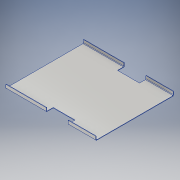
# Autodesk Inventor part: BellyPan
Saved by Autodesk Inventor 2016 (Build 200138000, 138)
## iProperties
Created: 2017-01-21
Part Number: BellyPan
Material: Aluminum 6061
Document SubType Name: Modeling
Designer: hamblettk
Density: 2.7 g/cm^3
Appearance: Aluminum - Flat
Author: hamblettk
Autodesk Inventor part; units mm, degrees
ref_plane "YZ Plane" through (0, 0, 0) normal (1, 0, 0) x (0, 1, 0)
ref_plane "XZ Plane" through (0, 0, 0) normal (0, 1, 0) x (-1, 0, 0)
ref_plane "XY Plane" through (0, 0, 0) normal (0, 0, 1) x (1, 0, 0)
sketch "Sketch2" plane through (0, 0, 0) normal (1, 0, 0) x (0, 1, 0)
  line L0 (0, 0) -> (0, -269.875)
  line L1 (0, 0) -> (0, 269.875)
  line L2 (0, 269.875) -> (25.4, 269.875)
  line L3 (0, -269.875) -> (25.4, -269.875)
  line L4 (25.4, -269.875) -> (25.4, -266.7)
  line L5 (25.4, 269.875) -> (25.4, 266.7)
  line L6 (25.4, 266.7) -> (3.175, 266.7)
  line L7 (25.4, -266.7) -> (3.175, -266.7)
  line L8 (3.175, -266.7) -> (3.175, 266.7)
  dimension "d10" = 269.875
  dimension "d11" = 269.875
  dimension "d12" = 25.4
  dimension "d13" = 25.4
  dimension "d14" = 3.175
  dimension "d15" = 3.175
  dimension "d16" = 22.225
  dimension "d17" = 22.225
  constraints: 18 end point, 4 vertical, 3 horizontal, 1 perpendicular
  measures "d10" distance of L0.start L0.end
  measures "d11" distance of L0.start L1.end
  measures "d12" distance of L1.end L2.end
  measures "d13" distance of L0.end L3.end
  measures "d14" distance of L3.end L4.end
  measures "d15" distance of L2.end L5.end
  measures "d16" distance of L5.end L6.end
  measures "d17" distance of L4.end L7.end
extrude "Extrusion2" add sketch "Sketch2" along normal blind 616.1532
fillet "Fillet1" radius 3.175 4 edges at (308.0766, 0, 269.875) (308.0766, 0, -269.875) (308.0766, 3.175, -266.7) (308.0766, 3.175, 266.7)
sketch "Sketch5" plane through (616.1532, 0, 0) normal (1, 0, 0) x (0, 0, -1)
  arc A0 (-269.875, 3.175) -> (-266.7, 0) centre (-266.7, 3.175) ccw projected
  line L0 (-266.7, 0) -> (-266.7, 3.175)
  line L1 (263.525, 3.175) -> (-263.525, 3.175) projected
  line L2 (-266.7, 3.175) -> (263.525, 3.175)
  line L3 (263.525, 3.175) -> (263.525, 0)
  line L4 (-266.7, 0) -> (266.7, 0) projected
  line L5 (263.525, 0) -> (-266.7, 0)
  point P0 (0, 0)
  constraints: 8 end point, 1 collinear, 1 horizontal, 1 perpendicular, 1 point on line, 1 tangent, 1 vertical
extrude "Extrusion6" add sketch "Sketch5" along normal blind 7.112
sketch "Sketch6" plane through (616.1532, 0, 0) normal (1, 0, 0) x (0, 0, -1)
  line L0 (-266.7, 6.35) -> (-266.7, 25.4) projected
  line L1 (-266.7, 25.4) -> (-269.875, 25.4) projected
  line L2 (-269.875, 25.4) -> (-269.875, 3.175) projected
  line L3 (-266.7, 3.175) -> (-263.525, 3.175) projected
  arc A0 (-266.7, 6.35) -> (-263.525, 3.175) centre (-263.525, 6.35) ccw projected
  line L4 (-266.7, 6.35) -> (-266.7, 25.4) projected
  line L5 (-266.7, 25.4) -> (-269.875, 25.4) projected
  line L6 (-269.875, 25.4) -> (-269.875, 3.175) projected
  arc A1 (-269.875, 3.175) -> (-266.7, 0) centre (-266.7, 3.175) ccw projected
  line L7 (-266.7, 0) -> (-266.7, 3.175) projected
  line L8 (263.525, 3.175) -> (263.525, 0) projected
  line L9 (263.525, 0) -> (266.7, 0) projected
  arc A2 (266.7, 0) -> (269.875, 3.175) centre (266.7, 3.175) ccw projected
  line L10 (269.875, 3.175) -> (269.875, 25.4) projected
  line L11 (269.875, 25.4) -> (266.7, 25.4) projected
  line L12 (266.7, 25.4) -> (266.7, 6.35) projected
  arc A3 (263.525, 3.175) -> (266.7, 6.35) centre (263.525, 6.35) ccw projected
  point P0 (0, 0)
extrude "Extrusion8" add sketch "Sketch6" along normal blind 3.937
sketch "Sketch7" plane through (0, 3.175, 263.525) normal (0, 1, 0) x (1, 0, 0)
  line L0 (0, 527.05) -> (620.0902, 527.05) projected
  line L1 (620.0902, 527.05) -> (429.9204, 527.05)
  line L2 (429.9204, 527.05) -> (277.5204, 527.05)
  line L3 (0, 263.525) -> (616.1532, 263.525)
  line L4 (623.2652, 527.05) -> (623.2652, -3.175) projected
  line L5 (0, 263.525) -> (616.1532, 263.525) construction
  line L6 (0, 0) -> (620.0902, 0)
  line L7 (277.5204, 0) -> (277.5204, 41.275)
  line L8 (277.5204, 41.275) -> (429.9204, 41.275)
  line L9 (429.9204, 41.275) -> (429.9204, 0)
  line L10 (277.5204, 527.05) -> (277.5204, 485.775)
  line L11 (429.9204, 527.05) -> (429.9204, 485.775)
  line L12 (429.9204, 485.775) -> (277.5204, 485.775)
  dimension "d38" = 190.1698
  dimension "d39" = 152.4
  dimension "d42" = 616.1532
  dimension "d43" = 0
  dimension "d48" = 152.4
  dimension "d50" = 41.275
  dimension "d51" = 41.275
  dimension "d52" = 41.275
  constraints: 22 end point, 4 point on line, 4 symmetric about line, 2 vertical, 1 collinear, 1 horizontal, 1 perpendicular
  measures "d38" distance of L0.end L1.end
  measures "d39" distance of L1.end L2.end
  measures "d42" distance of L3.start L3.end
  measures "d43" distance between parallel lines of L3 L5
  measures "d48" distance of L8.start L8.end
  measures "d50" distance of L2.end L10.end
  measures "d51" distance of L1.end L11.end
  measures "d52" distance of L7.start L8.start
extrude "Extrusion10" cut sketch "Sketch7" against normal blind 3.937
sketch "Sketch9" plane through (277.5204, 0, -263.525) normal (0, 0, 1) x (1, 0, 0)
  line L0 (0, 0) -> (0, 25.4)
  line L1 (-277.5204, 25.4) -> (342.5698, 25.4) projected
  line L2 (0, 25.4) -> (152.4, 25.4)
  line L3 (152.4, 3.175) -> (152.4, 0) projected
  line L4 (342.5698, 0) -> (-277.5204, 0) projected
  line L5 (152.4, 25.4) -> (152.4, 0)
  line L6 (152.4, 0) -> (0, 0) projected
  line L7 (152.4, 0) -> (0, 0)
  dimension "d55" = 152.4
  constraints: 8 end point, 2 point on line, 1 collinear, 1 vertical
  measures "d55" distance of L0.end L2.end
extrude "Extrusion11" cut sketch "Sketch9" against normal blind 6.35
sketch "Sketch10" plane through (429.9204, 0, 263.525) normal (0, 0, -1) x (-1, 0, 0)
  line L0 (152.4, 0) -> (152.4, 25.4)
  line L1 (429.9204, 25.4) -> (-190.1698, 25.4) projected
  line L2 (152.4, 25.4) -> (0, 25.4)
  line L3 (0, 25.4) -> (0, 0)
  line L4 (429.9204, 0) -> (-190.1698, 0) projected
  line L5 (0, 0) -> (152.4, 0)
  dimension "d58" = 25.4
  dimension "d59" = 152.4
  dimension "d60" = 25.4
  dimension "d61" = 152.4
  constraints: 8 end point, 2 point on line, 1 perpendicular
  measures "d58" distance of L0.start L0.end
  measures "d59" distance of L0.end L2.end
  measures "d60" distance of L2.end L3.end
  measures "d61" distance of L3.end L0.start
extrude "Extrusion12" cut sketch "Sketch10" against normal blind 6.35
sketch "Sketch11" plane through (277.5204, 3.175, -222.25) normal (1, 0, 0) x (0, 0, -1)
  line L0 (44.45, -3.175) -> (0, -3.175) projected
  arc A0 (44.45, -3.175) -> (47.625, 0) centre (44.45, 0) ccw projected
  line L1 (47.625, 22.225) -> (47.625, 0) projected
  line L2 (44.45, 22.225) -> (47.625, 22.225) projected
  line L3 (44.45, 3.175) -> (44.45, 22.225) projected
  arc A1 (41.275, 0) -> (44.45, 3.175) centre (41.275, 3.175) ccw projected
  line L4 (0, 0) -> (41.275, 0) projected
  line L5 (0, 0) -> (0, -3.175) projected
  line L6 (-444.5, -3.175) -> (-488.95, -3.175) projected
  line L7 (-444.5, 0) -> (-444.5, -3.175) projected
  line L8 (-485.775, 0) -> (-444.5, 0) projected
  arc A2 (-488.95, 3.175) -> (-485.775, 0) centre (-485.775, 3.175) ccw projected
  line L9 (-488.95, 22.225) -> (-488.95, 3.175) projected
  line L10 (-492.125, 22.225) -> (-488.95, 22.225) projected
  line L11 (-492.125, 0) -> (-492.125, 22.225) projected
  arc A3 (-492.125, 0) -> (-488.95, -3.175) centre (-488.95, 0) ccw projected
  point P0 (-222.25, -3.175)
extrude "Extrusion13" add sketch "Sketch11" along normal blind 2.0066
sketch "Sketch12" plane through (429.9204, 3.175, -263.525) normal (-1, 0, 0) x (0, 0, 1)
  line L0 (41.275, -3.175) -> (-3.175, -3.175) projected
  line L1 (41.275, 0) -> (41.275, -3.175) projected
  line L2 (0, 0) -> (41.275, 0) projected
  arc A0 (-3.175, 3.175) -> (0, 0) centre (0, 3.175) ccw projected
  line L3 (-3.175, 22.225) -> (-3.175, 3.175) projected
  line L4 (-6.35, 22.225) -> (-3.175, 22.225) projected
  line L5 (-6.35, 0) -> (-6.35, 22.225) projected
  arc A1 (-6.35, 0) -> (-3.175, -3.175) centre (-3.175, 0) ccw projected
  line L6 (530.225, -3.175) -> (485.775, -3.175) projected
  arc A2 (530.225, -3.175) -> (533.4, 0) centre (530.225, 0) ccw projected
  line L7 (533.4, 22.225) -> (533.4, 0) projected
  line L8 (530.225, 22.225) -> (533.4, 22.225) projected
  line L9 (530.225, 3.175) -> (530.225, 22.225) projected
  arc A3 (527.05, 0) -> (530.225, 3.175) centre (527.05, 3.175) ccw projected
  line L10 (485.775, 0) -> (527.05, 0) projected
  line L11 (485.775, 0) -> (485.775, -3.175) projected
  point P0 (263.525, -3.175)
extrude "Extrusion14" cut sketch "Sketch12" against normal blind 2.0066 contours L0 A1 L5 L4 L3 A0 L2 L1
body "Solid2"
